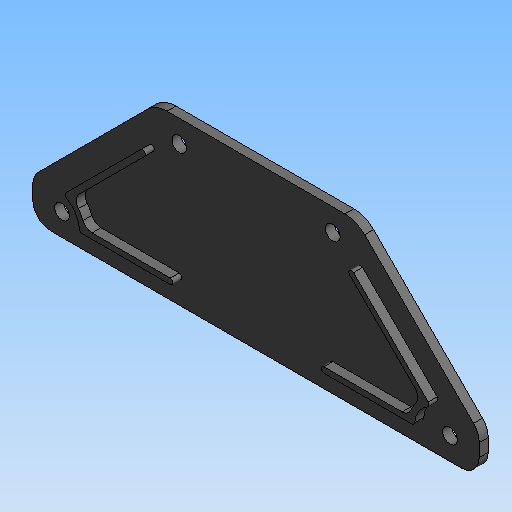
# Autodesk Inventor part: SWIVEL-HSMCS50
Saved by Autodesk Inventor 2020 (Build 240168000, 168)
## iProperties
Part Number: SWIVEL-HSMCS50
Material: 一般
Catalog Web Link: www.cadenas.de
Description: HSMC-SWIVEL-Casters for Aluminum Frames-Corner Angle Type
Vendor: MISUMI
Document SubType Name: Modeling
Designer: partserver
Manufacturer: MISUMI
Mass: 24.1952 g
Surface Area: 169.181 cm^2
Volume: 24.1952 cm^3
Density: 1 g/cm^3
Appearance: PSOLRGB-128-128-128
Category: PARTsolutions
Company: MISUMI
PSOL_IDENT_0: {$CADENAS_DATA\23d-libs\misumi\metric\39_accessories_for_al_extrusions\hsmc_swivel.prj},173 {VTYP=3D
PSOL_IDENT_1: },{NB=SWIVEL-HSMCS50},{LINA=SWIVEL-HSMCS50},{NN=HSMC-SWIVEL},{DATE=30.06.2021 13:18:54},{GEOMDATE=19
PSOL_IDENT_2: .12.2007 08:00:00},{VERSION=},{LINEID=60},{WBVAR=},{WBNUMERIC=}  {NB=SWIVEL-HSMCS50},{LINA=SWIVEL-HS
PSOL_IDENT_3: MCS50},{KT=DUMMY},{D=50},{TYPE=HSMCS},{AF=HFS5-2020},{H=70},{B=28},{DD=5.3},{E=27},{PN=SWIVEL-HSMCS5
PSOL_IDENT_4: 0}
NB: SWIVEL-HSMCS50
NN: HSMC-SWIVEL
NT: Casters for Aluminum Frames-Corner Angle Type
NBSYN: $PN.
LINA: SWIVEL-HSMCS50
CATALOG: Misumi
D: 50
TYPE: HSMCS
AF: HFS5-2020
H: 70
B: 28
DD: 5.3
E: 27
SUPPLIER: MISUMI
ARTICLENO: SWIVEL-HSMCS50
BOMINFO: SWIVEL-HSMCS50
CREATOR: CADENAS GmbH
Title: SWIVEL-HSMCS50
Author: Cadenas PARTsolutions
Comments: Casters for Aluminum Frames-Corner Angle Type
Autodesk Inventor part; units mm, degrees
sketch "Sketch_1" plane through (0, 0, 0) normal (0, 1, 0) x (-1, 0, 0)
  arc A0 (80, 22.5) -> (73.5, 29) centre (73.5, 22.5) ccw
  line L0 (73.5, 29) -> (-73.5, 29)
  arc A1 (-73.5, 29) -> (-80, 22.5) centre (-73.5, 22.5) ccw
  line L1 (-80, 22.5) -> (-80, 17.8995)
  arc A2 (-80, 17.8995) -> (-77.9497, 12.9497) centre (-73, 17.8995) ccw
  line L2 (-77.9497, 12.9497) -> (-38.9289, -26.0711)
  arc A3 (-38.9289, -26.0711) -> (-31.8579, -29) centre (-31.8579, -19) ccw
  line L3 (-31.8579, -29) -> (31.8579, -29)
  arc A4 (31.8579, -29) -> (38.9289, -26.0711) centre (31.8579, -19) ccw
  line L4 (38.9289, -26.0711) -> (77.9497, 12.9497)
  arc A5 (77.9497, 12.9497) -> (80, 17.8995) centre (73, 17.8995) ccw
  line L5 (80, 17.8995) -> (80, 22.5)
  circle A6 centre (-69.5, 21) radius 2.65
  circle A7 centre (-27.5, -21) radius 2.65
  circle A8 centre (27.5, -21) radius 2.65
  circle A9 centre (69.5, 21) radius 2.65
  constraints: 12 end point, 12 point on circle, 10 centre point
extrude "Extrusion1" add sketch "Sketch_1" along normal blind 3.2
sketch "Sketch_2" plane through (0, 0, 0) normal (0, 1, 0) x (-1, 0, 0)
  arc A0 (64.9121, 11.2258) -> (64.7093, 12.7964) centre (64.205, 11.9329) ccw
  arc A1 (60.0432, 20.0952) -> (64.7093, 12.7964) centre (69.5, 21) ccw
  arc A2 (60.0432, 20.0952) -> (59.0477, 21) centre (59.0477, 20) ccw
  line L0 (59.0477, 21) -> (27.5, 21)
  arc A3 (27.5, 21) -> (27.5, 19) centre (27.5, 20) ccw
  line L1 (27.5, 19) -> (55.5447, 19)
  arc A4 (58.8009, 16.7833) -> (55.5447, 19) centre (55.5447, 15.5) ccw
  arc A5 (58.8009, 16.7833) -> (60.4356, 13.9228) centre (69.5, 21) ccw
  arc A6 (60.1518, 9.2939) -> (60.4356, 13.9228) centre (57.6769, 11.7688) ccw
  line L2 (60.1518, 9.2939) -> (36.7378, -14.1201)
  arc A7 (36.7378, -14.1201) -> (38.152, -15.5343) centre (37.4449, -14.8272) ccw
  line L3 (38.152, -15.5343) -> (64.9121, 11.2258)
  constraints: 16 point on circle, 8 centre point, 8 end point
extrude "Extrusion2" add sketch "Sketch_2" against normal blind 3.2
sketch "Sketch_3" plane through (0, 0, 0) normal (0, 1, 0) x (-1, 0, 0)
  arc A0 (-27.5, 19) -> (-27.5, 21) centre (-27.5, 20) ccw
  line L0 (-27.5, 21) -> (-59.0477, 21)
  arc A1 (-59.0477, 21) -> (-60.0432, 20.0952) centre (-59.0477, 20) ccw
  arc A2 (-64.7093, 12.7964) -> (-60.0432, 20.0952) centre (-69.5, 21) ccw
  arc A3 (-64.7093, 12.7964) -> (-64.9121, 11.2258) centre (-64.205, 11.9329) ccw
  line L1 (-64.9121, 11.2258) -> (-38.152, -15.5343)
  arc A4 (-38.152, -15.5343) -> (-36.7378, -14.1201) centre (-37.4449, -14.8272) ccw
  line L2 (-36.7378, -14.1201) -> (-60.1518, 9.2939)
  arc A5 (-60.4356, 13.9228) -> (-60.1518, 9.2939) centre (-57.6769, 11.7688) ccw
  arc A6 (-60.4356, 13.9228) -> (-58.8009, 16.7833) centre (-69.5, 21) ccw
  arc A7 (-55.5447, 19) -> (-58.8009, 16.7833) centre (-55.5447, 15.5) ccw
  line L3 (-55.5447, 19) -> (-27.5, 19)
  constraints: 16 point on circle, 8 centre point, 8 end point
extrude "Extrusion3" add sketch "Sketch_3" against normal blind 3.2
ref_plane "swivel_to_body_XY" through (0, -3.2, 0) normal (0, 1, 0) x (1, 0, 0)
ref_plane "swivel_to_body_YZ" through (0, -3.2, 0) normal (1, 0, 0) x (0, 0, -1)
ref_plane "swivel_to_body_ZX" through (0, -3.2, 0) normal (0, 0, -1) x (0, 1, 0)
ref_plane "swivel_to_dummy_XY" through (0, 3.2, 0) normal (0, -1, 0) x (1, 0, 0)
ref_plane "swivel_to_dummy_YZ" through (0, 3.2, 0) normal (1, 0, 0) x (0, 0, 1)
ref_plane "swivel_to_dummy_ZX" through (0, 3.2, 0) normal (0, 0, 1) x (0, -1, 0)
body "Solid1"
